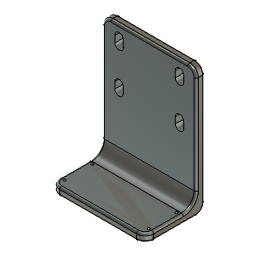
Polycase-Voltaic-Bracket v7 (Autodesk Fusion 360 design; units mm, degrees)
Autodesk Fusion 360 part; units mm, degrees
sketch "Sketch1" plane through (0, 0, 0) normal (0, 0, 1) x (1, 0, 0)
sketch "Sketch2" plane through (0, 0, 0) normal (0, 0, 1) x (1, 0, 0)
  line L0 (-101.7193, 55.502) -> (37.9807, 55.502)
  line L1 (37.9807, 55.502) -> (37.9807, -33.398)
  line L2 (37.9807, -33.398) -> (-101.7193, -33.398)
  line L3 (-101.7193, -33.398) -> (-101.7193, 55.502)
  dimension "d1" = 139.7
  dimension "d2" = 88.9
  constraint horizontal L0
  constraint vertical L1
  constraint horizontal L2
  constraint vertical L3
  measures "d1" distance of L0.start L0.end
  measures "d2" distance of L0.end L1.end
extrude "Extrude1" add sketch "Sketch2" along normal blind 12.7
sketch "Sketch3" plane through (0, 0, 12.7) normal (0, 0, 1) x (-1, 0, 0)
  line L0 (101.7193, 33.398) -> (-37.9807, 33.398)
  line L1 (-37.9807, 33.398) -> (-37.9807, -55.502)
  line L2 (-37.9807, -55.502) -> (101.7193, -55.502)
  line L3 (101.7193, -55.502) -> (101.7193, 33.398)
sketch "Sketch4" plane through (0, 0, 12.7) normal (0, 0, 1) x (-1, 0, 0)
  line L0 (-37.9807, -55.502) -> (101.7193, -55.502)
  line L1 (101.7193, -55.502) -> (101.7193, -42.802)
  line L2 (101.7193, -42.802) -> (-37.9807, -42.802)
  line L3 (-37.9807, -42.802) -> (-37.9807, -55.502)
  line L4 (101.7193, -55.502) -> (101.7193, 33.398)
  point P0 (-37.9807, -55.502)
  dimension "d5" = 12.7
  constraint horizontal L0
  constraint vertical L1
  constraint horizontal L2
  constraint vertical L3
  constraint coincident L1.end L4
  constraint coincident P0 L0.start
  measures "d5" distance of L0.end L1.end
extrude "Extrude2" add sketch "Sketch4" along normal blind 177.8
fillet "Fillet1" radius 19.05 1 edges at (-31.8693, 42.802, 12.7)
sketch "Sketch5" plane through (0, 0, 0) normal (0, 0, -1) x (1, 0, 0)
  line L0 (37.9807, 33.398) -> (-101.7193, 33.398)
  line L1 (-101.7193, 33.398) -> (-101.7193, -55.502)
  line L2 (-101.7193, -55.502) -> (37.9807, -55.502)
  line L3 (37.9807, -55.502) -> (37.9807, 33.398)
  line L4 (-94.5819, 33.398) -> (-94.5819, 20.698) construction
  line L5 (-94.5819, 20.698) -> (-101.7193, 20.698) construction
  line L6 (30.8433, 33.398) -> (30.8433, 20.698) construction
  line L7 (30.8433, 20.698) -> (37.9807, 20.698) construction
  line L8 (-94.5819, 20.698) -> (-94.5819, -20.577) construction
  line L9 (-94.5819, -20.577) -> (30.8433, -20.577) construction
  line L10 (30.8433, -20.577) -> (30.8433, 20.698) construction
  line L11 (-94.5819, 20.698) -> (30.8433, 20.698) construction
  circle A0 centre (-94.5819, 20.698) radius 1.905
  circle A1 centre (30.8433, 20.698) radius 1.905
  circle A2 centre (30.8433, -20.577) radius 1.905
  circle A3 centre (-94.5819, -20.577) radius 1.905
  dimension "d12" = 41.275
  dimension "d13" = 125.4252
  dimension "d14" = 3.81
  dimension "d15" = 12.7
  constraint coincident L0 L4.start
  constraint perpendicular L0 L4
  constraint coincident L1 L5.end
  constraint perpendicular L1 L5
  constraint coincident L0 L6.start
  constraint perpendicular L0 L6
  constraint coincident L3 L7.end
  constraint perpendicular L3 L7
  constraint collinear L5 L7
  constraint equal L5 L7
  constraint perpendicular L5 L8
  constraint perpendicular L6 L9
  constraint perpendicular L7 L10
  constraint coincident L4.end L5.start
  constraint coincident L6.end L7.start
  constraint coincident L9.end L10.start
  constraint coincident L8.end L9.start
  constraint equal A1 A2
  constraint equal A2 A3
  constraint equal A0 A3
  measures "d12" distance of L4.end L8.end
  measures "d13" distance of L4.end L6.end
  measures "d14" diameter of A0
  measures "d15" distance of L4.start L4.end
extrude "Extrude3" cut sketch "Sketch5" against normal through all contours A0 | A1 | A2 | A3
fillet "Fillet2" radius 12.7 2 edges at (37.9807, -33.398, 6.35) (-101.7193, -33.398, 6.35)
fillet "Fillet3" radius 3.175 18 edges at (37.9807, 17.402, 0) (34.2609, -29.6782, 0) (-31.8693, -33.398, 0) (-97.9996, -29.6782, 0) (-101.7193, 17.402, 0) (37.9807, 42.802, 111.125) (37.9807, 37.2224, 18.2796) (37.9807, 1.527, 12.7) (34.2609, -29.6782, 12.7) (-31.8693, -33.398, 12.7) (-97.9996, -29.6782, 12.7) (-101.7193, 1.527, 12.7) (-101.7193, 37.2224, 18.2796) (-101.7193, 42.802, 111.125) (-101.7193, 55.502, 95.25) (-31.8693, 42.802, 190.5) (-31.8693, 55.502, 190.5) (37.9807, 55.502, 95.25)
fillet "Fillet4" radius 12.7 3 edges at (-100.7894, 54.5721, 0.9299) (-31.8693, 55.502, 0) (37.0507, 54.5721, 0.9299)
sketch "Sketch6" plane through (0, 42.802, 0) normal (0, -1, 0) x (1, 0, 0)
  line L0 (34.8057, 31.75) -> (34.8057, 187.325)
  line L1 (34.8057, 187.325) -> (-98.5443, 187.325)
  line L2 (-98.5443, 187.325) -> (-98.5443, 31.75)
  line L3 (-98.5443, 31.75) -> (34.8057, 31.75)
fillet "Fillet5" radius 12.7 6 edges at (-100.7894, 54.5721, 189.5701) (-101.7193, 49.152, 190.5) (-100.7894, 43.732, 189.5701) (37.0507, 43.732, 189.5701) (37.9807, 49.152, 190.5) (37.0507, 54.5721, 189.5701)
sketch "Sketch7" plane through (0, 55.502, 0) normal (0, 1, 0) x (-1, 0, 0)
  arc A0 (-25.2807, 187.325) -> (-34.8057, 177.8) centre (-25.2807, 177.8) ccw
  line L0 (-34.8057, 177.8) -> (-34.8057, 12.7)
  line L1 (-34.8057, 12.7) -> (98.5443, 12.7)
  line L2 (98.5443, 12.7) -> (98.5443, 177.8)
  arc A1 (98.5443, 177.8) -> (89.0193, 187.325) centre (89.0193, 177.8) ccw
  line L3 (89.0193, 187.325) -> (-25.2807, 187.325)
  line L4 (-34.8057, 173.075) -> (-13.1357, 173.075) construction
  line L5 (-13.1357, 173.075) -> (-13.1357, 187.325) construction
  line L6 (76.8743, 187.325) -> (76.8743, 173.075) construction
  line L7 (76.8743, 173.075) -> (98.5443, 173.075) construction
  line L8 (-6.8857, 173.075) -> (76.8743, 173.075) construction
  line L9 (-13.1357, 173.075) -> (-13.1357, 163.575) construction
  line L10 (76.8743, 173.075) -> (76.8743, 163.575) construction
  line L11 (-13.1357, 163.575) -> (-6.8857, 163.575) construction
  line L12 (-6.8857, 173.075) -> (-19.3857, 173.075) construction
  line L13 (-19.3857, 163.5751) -> (-19.3857, 173.075)
  line L14 (-6.8857, 173.075) -> (-6.8857, 163.575)
  arc A2 (-6.8857, 173.075) -> (-19.3857, 173.075) centre (-13.1357, 173.075) ccw
  arc A3 (-19.3857, 163.5751) -> (-6.8857, 163.575) centre (-13.1357, 163.575) ccw
  line L15 (70.6243, 173.075) -> (70.6243, 163.575)
  line L16 (83.1238, 163.495) -> (83.0355, 173.075)
  arc A4 (70.6243, 163.575) -> (83.1238, 163.495) centre (76.8743, 163.575) ccw
  arc A5 (83.0355, 173.075) -> (70.6243, 173.075) centre (76.8299, 173.8189) ccw
  line L17 (-13.1357, 163.575) -> (-13.1357, 113.575) construction
  line L18 (76.8743, 163.575) -> (76.8743, 113.575)
  line L19 (-13.1357, 113.575) -> (-13.1357, 104.075) construction
  line L20 (76.8743, 113.575) -> (76.8743, 104.075) construction
  line L21 (-13.1357, 104.075) -> (-6.8857, 104.075) construction
  line L22 (-6.8857, 113.5783) -> (-6.8857, 104.075)
  line L23 (-19.3857, 104.0732) -> (-19.3857, 113.575)
  arc A6 (-6.8857, 113.5783) -> (-19.3857, 113.575) centre (-13.1357, 113.575) ccw
  arc A7 (-19.3857, 104.0732) -> (-6.8857, 104.075) centre (-13.1357, 104.075) ccw
  line L24 (76.8743, 113.575) -> (70.6243, 113.575) construction
  line L25 (70.6243, 113.575) -> (70.6243, 104.075)
  line L26 (76.8743, 113.575) -> (83.1243, 113.575) construction
  line L27 (83.1243, 113.575) -> (83.1243, 104.075)
  arc A8 (83.1243, 113.575) -> (70.6243, 113.575) centre (76.8743, 113.575) ccw
  arc A9 (70.6243, 104.075) -> (83.1243, 104.075) centre (76.8743, 104.075) ccw
  dimension "d25" = 90.01
  dimension "d26" = 14.25
  dimension "d27" = 12.5
  dimension "d28" = 23.75
  dimension "d29" = 9.5
  dimension "d30" = 12.5
  dimension "d33" = 6.25
  dimension "d34" = 50
  constraint coincident L0 L4.start
  constraint perpendicular L0 L4
  constraint coincident L3 L5.end
  constraint perpendicular L3 L5
  constraint coincident L3 L6.start
  constraint perpendicular L3 L6
  constraint coincident L2 L7.end
  constraint perpendicular L2 L7
  constraint equal L4 L7
  constraint equal L5 L6
  constraint coincident L4.end L5.start
  constraint perpendicular L4 L9
  constraint perpendicular L7 L10
  constraint equal L9 L10
  constraint coincident L9.end L11.start
  constraint coincident L10.end A4.centre
  constraint equal A3 A4
  constraint equal A2 A3
  constraint perpendicular L9 L11
  constraint coincident L4 L12.end
  constraint tangent L13 A2
  constraint coincident L8 L15.start
  constraint tangent L15 A4
  constraint perpendicular L8 L15
  constraint coincident L7 L16.end
  constraint perpendicular L11 L17
  constraint perpendicular L8 L18
  constraint equal L17 L18
  constraint coincident L17.end L19.start
  constraint coincident L18.end L20.start
  constraint parallel L17 L19
  constraint parallel L18 L20
  constraint equal L19 L20
  constraint coincident L19.end L21.start
  constraint coincident L20.end A9.centre
  constraint equal A6 A7
  constraint equal A6 A8
  constraint equal A8 A9
  constraint perpendicular L19 L21
  constraint tangent L22 A7
  constraint tangent L23 A6
  constraint perpendicular L21 L23
  constraint perpendicular L18 L24
  constraint tangent L25 A9
  constraint perpendicular L18 L26
  constraint tangent L27 A9
  constraint horizontal L8
  measures "d25" distance of L4.end L6.end
  measures "d26" distance of L4.end L5.end
  measures "d27" diameter of A2
  measures "d28" distance of L3 L9.end
  measures "d29" distance of L17.end L19.end
  measures "d30" diameter of A6
  measures "d33" radius of A5
  measures "d34" distance of L9.end L17.end
extrude "Extrude4" cut sketch "Sketch7" against normal through all contours L13 L14 A2 A3 | L15 L16 A4 A5 | L22 L23 A6 A7 | L25 L27 A8 A9
